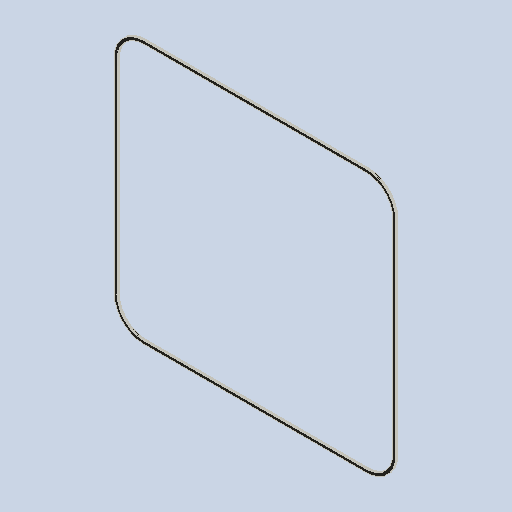
# Autodesk Inventor part: Caucho
Saved by Autodesk Inventor 2022.4 (Build 264492000, 492)
## iProperties
Created: 2022-11-28
Part Number: Caucho
Material: Generic
Document SubType Name: Sheet Metal
Designer: David
Density: 1 g/cm^3
Sheet Metal Rule: Default
Appearance: Gunmetal
Author: David
Autodesk Inventor part; units mm, degrees
ref_plane "YZ Plane" through (0, 0, 0) normal (1, 0, 0) x (0, 1, 0)
ref_plane "XZ Plane" through (0, 0, 0) normal (0, 1, 0) x (-1, 0, 0)
ref_plane "XY Plane" through (0, 0, 0) normal (0, 0, 1) x (1, 0, 0)
sketch "Sketch5" plane through (0, 0, 0) normal (0, 0, 1) x (1, 0, 0)
  line L0 (-900, -850) -> (900, -850)
  line L1 (900, -850) -> (900, 850)
  line L2 (900, 850) -> (-900, 850)
  line L3 (-900, 850) -> (-900, -850)
  line L4 (-900, -850) -> (900, 850) construction
  line L5 (900, -850) -> (-900, 850) construction
  line L6 (-600, 700) -> (600, 700)
  line L7 (750, 550) -> (750, -550)
  line L8 (600, -700) -> (-600, -700)
  line L9 (-750, -550) -> (-750, 550)
  arc A0 (750, 550) -> (600, 700) centre (600, 550) ccw
  arc A1 (-600, 700) -> (-750, 550) centre (-600, 550) ccw
  arc A2 (-750, -550) -> (-600, -700) centre (-600, -550) ccw
  arc A3 (600, -700) -> (750, -550) centre (600, -550) ccw
  line L10 (600, 697) -> (-600, 697)
  arc A4 (-600, 697) -> (-747, 550) centre (-600, 550) ccw
  line L11 (-747, 550) -> (-747, -550)
  arc A5 (-747, -550) -> (-600, -697) centre (-600, -550) ccw
  line L12 (-600, -697) -> (600, -697)
  arc A6 (600, -697) -> (747, -550) centre (600, -550) ccw
  line L13 (747, -550) -> (747, 550)
  arc A7 (747, 550) -> (600, 697) centre (600, 550) ccw
  point P0 (0, 0)
  point P1 (0, 0)
  dimension "d0" = 1800
  dimension "d1" = 1700
  dimension "d2" = 150
  dimension "d3" = 150
  dimension "d4" = 150
  dimension "d5" = 150
  dimension "d6" = 150
  dimension "d9" = 3
  constraints: 28 end point, 16 point on circle, 8 centre point, 8 tangent, 6 parallel, 3 perpendicular, 2 midpoint, 1 horizontal, 10 other
  measures "d0" distance of L2.end L1.end
  measures "d1" distance of L1.end L0.end
  measures "d2" distance between parallel lines of L2 L6
  measures "d3" radius of A0
  measures "d4" radius of A1
  measures "d5" radius of A2
  measures "d6" radius of A3
  measures "d9" distance between parallel lines of L6 L10
extrude "Extrusion1" add sketch "Sketch5" along normal mid plane 3.048 contours L6 A0 L7 A3 L8 A2 L9 A1
sketch "Sketch6" plane through (0, 0, 1.524) normal (0, 0, 1) x (1, 0, 0)
  line L0 (-600, -700) -> (600, -700) projected
  arc A0 (600, -700) -> (750, -550) centre (600, -550) ccw projected
  line L1 (750, -550) -> (750, 550) projected
  arc A1 (750, 550) -> (600, 700) centre (600, 550) ccw projected
  line L2 (600, 700) -> (-600, 700) projected
  arc A2 (-600, 700) -> (-750, 550) centre (-600, 550) ccw projected
  line L3 (-750, 550) -> (-750, -550) projected
  arc A3 (-750, -550) -> (-600, -700) centre (-600, -550) ccw projected
  arc A4 (747, 550) -> (600, 697) centre (600, 550) ccw projected
  line L4 (747, 550) -> (747, -550) projected
  arc A5 (600, -697) -> (747, -550) centre (600, -550) ccw projected
  line L5 (600, -697) -> (-600, -697) projected
  arc A6 (-747, -550) -> (-600, -697) centre (-600, -550) ccw projected
  line L6 (-747, -550) -> (-747, 550) projected
  arc A7 (-600, 697) -> (-747, 550) centre (-600, 550) ccw projected
  line L7 (-600, 697) -> (600, 697) projected
  line L8 (-600, 708) -> (600, 708)
  arc A8 (758, 550) -> (600, 708) centre (600, 550) ccw
  line L9 (758, 550) -> (758, -550)
  arc A9 (600, -708) -> (758, -550) centre (600, -550) ccw
  line L10 (600, -708) -> (-600, -708)
  arc A10 (-758, -550) -> (-600, -708) centre (-600, -550) ccw
  line L11 (-758, -550) -> (-758, 550)
  arc A11 (-600, 708) -> (-758, 550) centre (-600, 550) ccw
  arc A12 (741, 550) -> (600, 691) centre (600, 550) ccw
  line L12 (741, 550) -> (741, -550)
  arc A13 (600, -691) -> (741, -550) centre (600, -550) ccw
  line L13 (600, -691) -> (-600, -691)
  arc A14 (-741, -550) -> (-600, -691) centre (-600, -550) ccw
  line L14 (-741, -550) -> (-741, 550)
  arc A15 (-600, 691) -> (-741, 550) centre (-600, 550) ccw
  line L15 (-600, 691) -> (600, 691)
  point P0 (0, 0)
  dimension "d12" = 8
  dimension "d13" = 6
  constraints: 16 end point, 16 point on circle, 8 centre point, 14 other
  measures "d12" distance between parallel lines of L2 L8
  measures "d13" distance between parallel lines of L7 L15
extrude "Extrusion2" add sketch "Sketch6" along normal blind 4 contours A3 L3 A2 L2 A1 L1 A0 L0 | L4 A5 L5 A6 L6 A7 L7 A4 | L8 A8 L9 A9 L10 A10 L11 A11
sketch "Sketch7" plane through (0, 0, -1.524) normal (0, 0, -1) x (-1, 0, 0)
  line L0 (600, -708) -> (-600, -708) projected
  arc A0 (600, -708) -> (758, -550) centre (600, -550) ccw projected
  line L1 (758, 550) -> (758, -550) projected
  arc A1 (758, 550) -> (600, 708) centre (600, 550) ccw projected
  line L2 (-600, 708) -> (600, 708) projected
  arc A2 (-600, 708) -> (-758, 550) centre (-600, 550) ccw projected
  line L3 (-758, -550) -> (-758, 550) projected
  arc A3 (-758, -550) -> (-600, -708) centre (-600, -550) ccw projected
  arc A4 (600, -700) -> (750, -550) centre (600, -550) ccw projected
  line L4 (600, -700) -> (-600, -700) projected
  arc A5 (-750, -550) -> (-600, -700) centre (-600, -550) ccw projected
  line L5 (-750, -550) -> (-750, 550) projected
  arc A6 (-600, 700) -> (-750, 550) centre (-600, 550) ccw projected
  line L6 (-600, 700) -> (600, 700) projected
  arc A7 (750, 550) -> (600, 700) centre (600, 550) ccw projected
  line L7 (750, 550) -> (750, -550) projected
  line L8 (-600, -700) -> (600, -700) projected
  arc A8 (600, -700) -> (750, -550) centre (600, -550) ccw projected
  line L9 (750, -550) -> (750, 550) projected
  arc A9 (750, 550) -> (600, 700) centre (600, 550) ccw projected
  line L10 (600, 700) -> (-600, 700) projected
  arc A10 (-600, 700) -> (-750, 550) centre (-600, 550) ccw projected
  line L11 (-750, 550) -> (-750, -550) projected
  arc A11 (-750, -550) -> (-600, -700) centre (-600, -550) ccw projected
  arc A12 (-600, 697) -> (-747, 550) centre (-600, 550) ccw projected
  line L12 (-600, 697) -> (600, 697) projected
  arc A13 (747, 550) -> (600, 697) centre (600, 550) ccw projected
  line L13 (747, 550) -> (747, -550) projected
  arc A14 (600, -697) -> (747, -550) centre (600, -550) ccw projected
  line L14 (600, -697) -> (-600, -697) projected
  arc A15 (-747, -550) -> (-600, -697) centre (-600, -550) ccw projected
  line L15 (-747, -550) -> (-747, 550) projected
  line L16 (-600, -691) -> (600, -691) projected
  arc A16 (-741, -550) -> (-600, -691) centre (-600, -550) ccw projected
  line L17 (-741, 550) -> (-741, -550) projected
  arc A17 (-600, 691) -> (-741, 550) centre (-600, 550) ccw projected
  line L18 (600, 691) -> (-600, 691) projected
  arc A18 (741, 550) -> (600, 691) centre (600, 550) ccw projected
  line L19 (741, -550) -> (741, 550) projected
  arc A19 (600, -691) -> (741, -550) centre (600, -550) ccw projected
  line L20 (600, 697) -> (-600, 697) projected
  arc A20 (-600, 697) -> (-747, 550) centre (-600, 550) ccw projected
  line L21 (-747, 550) -> (-747, -550) projected
  arc A21 (-747, -550) -> (-600, -697) centre (-600, -550) ccw projected
  line L22 (-600, -697) -> (600, -697) projected
  arc A22 (600, -697) -> (747, -550) centre (600, -550) ccw projected
  line L23 (747, -550) -> (747, 550) projected
  arc A23 (747, 550) -> (600, 697) centre (600, 550) ccw projected
  point P0 (0, 0)
extrude "Extrusion3" add sketch "Sketch7" along normal blind 4 contours L0 A3 L3 A2 L2 A1 L1 A0 | L4 A5 L5 A6 L6 A7 L7 A4 | L12 A13 L13 A14 L14 A15 L15 A12
equation "\"d10\" = Thickness"
equation "\"BendRadius\" = Thickness"
equation "\"BendReliefWidth\" = Thickness"
equation "\"BendReliefDepth\" = 0.5 * Thickness"
equation "\"CornerReliefSize\" = 4 * Thickness"
equation "\"MinimumRemnant\" = 2 * Thickness"
equation "\"TransitionRadius\" = BendRadius"
equation "\"JacobiRadiusSize\" = BendRadius"
equation "\"GapSize\" = Thickness"
equation "\"Space6\" = 0"
equation "\"Space7\" = 0"
equation "\"Thickness\" = 3.048"
body "Solid1"
